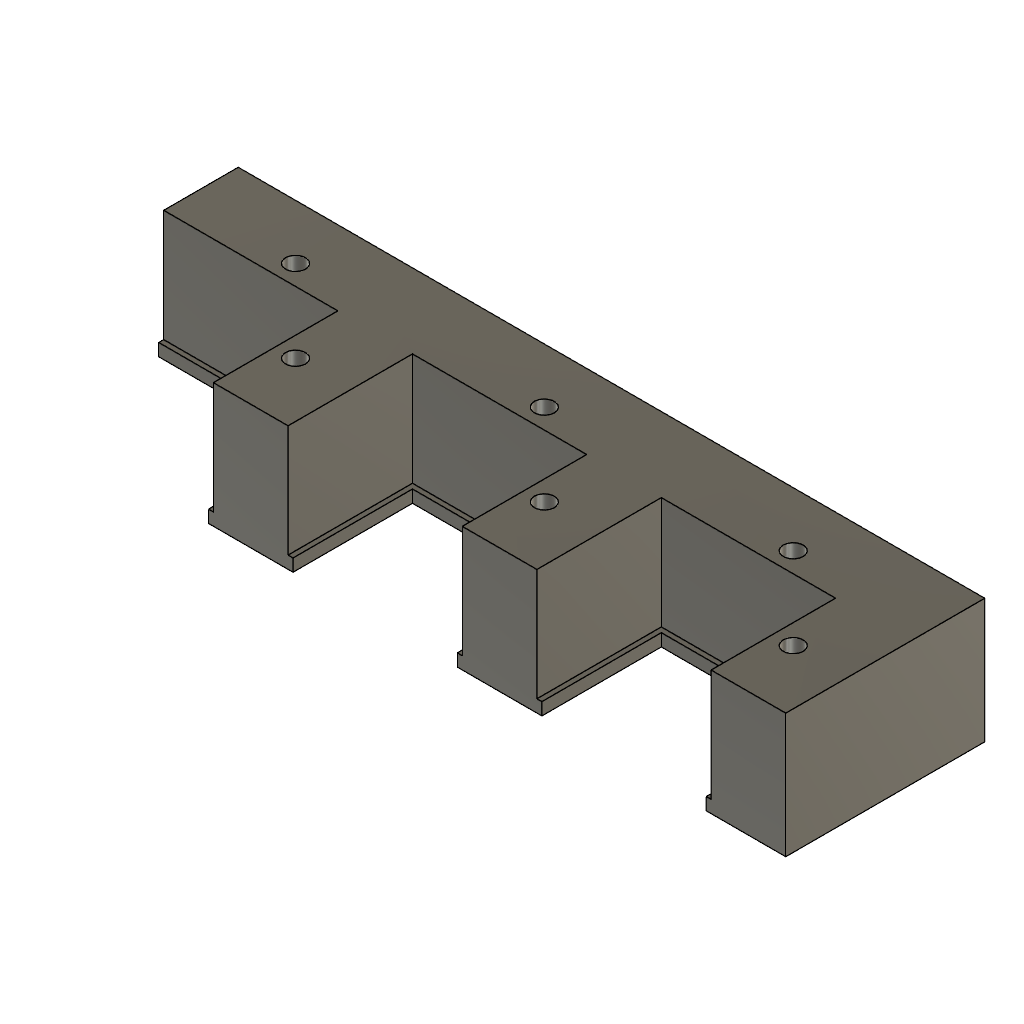
multi_cylinders20261002 (Autodesk Fusion 360 design; units mm, degrees)
Autodesk Fusion 360 part; units mm, degrees
sketch "スケッチ1" plane through (0, 0, 0) normal (0, 0, 1) x (1, 0, 0)
  circle A0 centre (-40, -40) radius 30
  circle A1 centre (-40, -40) radius 35
  line L0 (0, 0) -> (-80, 0)
  line L1 (-80, 0) -> (-80, -60)
  line L2 (-80, -60) -> (0, -60)
  line L3 (0, -60) -> (0, 0)
  line L4 (-80, -60) -> (-10, -60)
  line L5 (-10, -60) -> (-10, -10)
  line L6 (-10, -10) -> (-80, -10)
  line L7 (-80, -10) -> (-80, -60)
  line L8 (-80, -60) -> (-12, -60)
  line L9 (-12, -60) -> (-12, -12)
  line L10 (-12, -12) -> (-80, -12)
  line L11 (-80, -12) -> (-80, -60)
  line L12 (-80, 0) -> (0, 0)
  line L13 (20, 0) -> (20, 20)
  line L14 (20, 20) -> (-80, 20)
  line L15 (-80, 20) -> (-80, 0)
  line L16 (0, 0) -> (0, -60)
  line L17 (0, -60) -> (20, -60)
  line L18 (20, -60) -> (20, 0)
  line L19 (-80, -60) -> (-78, -60)
  line L20 (-78, -60) -> (-78, 0)
  line L21 (-78, 0) -> (-80, 0)
  line L22 (-80, 0) -> (-80, -60)
  dimension "d1" = 60
  dimension "d2" = 70
  dimension "d4" = 60
  dimension "d5" = 70
  dimension "d6" = 50
  dimension "d9" = 68
  dimension "d10" = 48
  dimension "d13" = 80
  dimension "d14" = 100
  dimension "d15" = 20
  dimension "d29" = 2
  constraint concentric A0 A1
  constraint horizontal L0
  constraint vertical L1
  constraint horizontal L2
  constraint vertical L3
  constraint coincident L0.start L3.end
  constraint horizontal L4
  constraint vertical L5
  constraint horizontal L6
  constraint vertical L7
  constraint horizontal L8
  constraint vertical L9
  constraint horizontal L10
  constraint vertical L11
  constraint horizontal L12
  constraint vertical L13
  constraint horizontal L14
  constraint vertical L15
  constraint vertical L16
  constraint horizontal L17
  constraint vertical L18
  constraint coincident L3 L0.start
  constraint tangent A0 L5
  constraint tangent A0 L6
  constraint horizontal L19
  constraint vertical L20
  constraint horizontal L21
  constraint vertical L22
  constraint coincident L12 L20.end
  measures "d1" diameter of A0
  measures "d2" diameter of A1
  measures "d4" distance of L0.start L2.end
  measures "d5" distance of L1.end L4.end
  measures "d6" distance of L1.end L6.end
  measures "d9" distance of L1.end L8.end
  measures "d10" distance of L1.end L10.end
  measures "d13" distance of L0.start L0.end
  measures "d14" distance of L0.end L13.start
  measures "d15" distance of L0.end L14.end
  measures "d29" distance of L1.end L19.end
extrude "押し出し1" add sketch "スケッチ1" along normal blind 50 contours A1 L5 | A1 L0 L2 L3 L5 L6 L12 L16 L20 | A1 L6 | L0 L1 L6 L12 L20 L21 L22 makes body 1
extrude "押し出し2" add sketch "スケッチ1" along normal blind 5 separate body contours A0 L9 | A0 A1 L2 L4 L5 L9 | A0 A1 L5 L9 | A1 L2 L4 L5 | A1 L5 L6 L9 L10 | A0 L10 | A0 A1 L6 L10 | A0 A1 L6 L10 | A1 L6 L10 L20 | L1 L2 L4 L7 L8 L10 L11 L19 L20 L22 | L1 L6 L7 L10 L20 L22 makes body 2
extrude "押し出し3" add sketch "スケッチ1" along normal blind 50 separate body contours L0 L3 L12 L13 L14 L15 L16 L17 L18 L21 makes body 3
copy_body "ボディのコピーと貼り付け1" bodies 1 2 3 makes body 4 makes body 5 makes body 6
combine "結合1" operation add target body 4 tool bodies 5 6
extrude "押し出し4" add sketch "スケッチ1" along normal blind 60 from surface at 5 separate body contours A0 L9 | A0 L2 L4 L8 L9 L10 | A0 L10 | A0 L2 L4 L8 makes body 7
copy_body "ボディのコピーと貼り付け2" bodies 4 7 makes body 8 makes body 9
sketch "スケッチ2" plane through (0, 0, 50) normal (0, 0, 1) x (-1, 0, 0)
  line L0 (10, 60) -> (-20, 60)
  line L1 (-20, 60) -> (-20, -20)
  line L2 (-20, -20) -> (80, -20)
  line L3 (80, -20) -> (80, 10)
  line L4 (80, 10) -> (10, 10)
  line L5 (10, 10) -> (10, 60)
  circle A0 centre (35, 2) radius 4
  circle A1 centre (2, 35) radius 4
  dimension "d21" = 8
  dimension "d22" = 8
  dimension "d23" = 8
  dimension "d24" = 8
  dimension "d25" = 45
  dimension "d26" = 25
  measures "d21" diameter of A0
  measures "d22" diameter of A1
  measures "d23" distance of L4 A0.centre
  measures "d24" distance of L5 A1.centre
  measures "d25" distance of L3 A0.centre
  measures "d26" distance of L0 A1.centre
extrude "押し出し5" cut sketch "スケッチ2" against normal blind 30 contours A0 | A1 bodies 1 3 4 8
copy_body "ボディのコピーと貼り付け3" bodies 8 9 makes body 10 makes body 11
move_body "移動1" bodies 10 11 to x (1, 0, 0) y (0, 1, 0) z (0, 0, 1) at (100, 0, 0)
copy_body "ボディのコピーと貼り付け4" bodies 8 9 makes body 12 makes body 13
move_body "移動2" bodies 12 13 to x (1, 0, 0) y (0, 1, 0) z (0, 0, 1) at (200, 0, 0)
combine "結合2" operation add target body 4 tool bodies 10 12
sketch "スケッチ3" plane through (0, 0, 0) normal (0, 0, 1) x (1, 0, 0)
  line L0 (-86.1051, -12) -> (-78, -12)
  line L1 (-78, -12) -> (-78, -61.0005)
  line L2 (-78, -61.0005) -> (-86.1051, -61.0005)
  line L3 (-86.1051, -61.0005) -> (-86.1051, -12)
  point P0 (-78, -12)
  constraint horizontal L0
  constraint vertical L1
  constraint horizontal L2
  constraint vertical L3
  constraint vertical P0 L0.end
  constraint coincident P0 L0.end
extrude "押し出し6" cut sketch "スケッチ3" along normal blind 10 bodies 4
copy_body "ボディのコピーと貼り付け5" bodies 4 makes body 14
copy_body "ボディのコピーと貼り付け6" bodies 4 makes body 15
sketch "スケッチ4" plane through (0, 0, 5) normal (0, 0, 1) x (-1, 0, 0)
  line L0 (80, 12) -> (12, 12)
  line L1 (12, 12) -> (12, 60)
  line L2 (12, 60) -> (10, 60)
  line L3 (10, 60) -> (10, 10)
  line L4 (10, 10) -> (80, 10)
  line L5 (80, 10) -> (80, 12)
  circle A0 centre (25, 25) radius 15
  circle A1 centre (-35, 25) radius 15
  circle A2 centre (-75, 25) radius 15
  line L6 (-20, 10) -> (-90, 10)
  line L7 (-20, 60) -> (-20, 10)
  line L8 (-90, 10) -> (-90, 60)
  circle A3 centre (-135, 25) radius 15
  circle A4 centre (-175, 25) radius 15
  dimension "d32" = 30
  dimension "d33" = 30
  dimension "d34" = 30
  dimension "d35" = 30
  dimension "d36" = 30
  constraint tangent L4 A0
  constraint tangent L3 A0
  constraint tangent A1 L6
  constraint tangent A1 L7
  constraint tangent A2 L6
  constraint tangent A2 L8
  measures "d32" diameter of A0
  measures "d33" diameter of A1
  measures "d34" diameter of A2
  measures "d35" diameter of A3
  measures "d36" diameter of A4
extrude "押し出し7" add sketch "スケッチ4" along normal blind 60 separate body contours A1 | A2 | A3 | A4 makes body 16 at (60.0745, -23.5065, 25) makes body 17 at (120.0745, -23.5065, 45) makes body 18 at (20.0745, -23.5065, 25) makes body 19 at (160.0745, -23.5065, 45)
